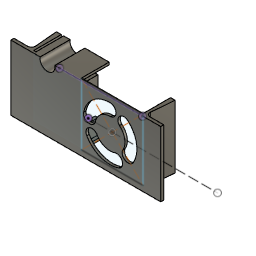
Tapa_fuente (Autodesk Fusion 360 design; units mm, degrees)
Autodesk Fusion 360 part; units mm, degrees
note: some values were not read from the file. Set by a fixed rule: which sketch regions a step uses.
sketch "Sketch1" plane through (0, 0, 0) normal (0, 1, 0) x (1, 0, 0)
  line L0 (38, -21) -> (-38, -21)
  line L1 (-38, -21) -> (-38, 21)
  line L2 (-38, 21) -> (38, 21)
  line L3 (38, 21) -> (38, -21)
  line L4 (38, -21) -> (-38, 21) construction
  line L5 (-38, -21) -> (38, 21) construction
  line L6 (-38, -21) -> (-50, -21)
  line L7 (-50, -21) -> (-50, 21)
  line L8 (-50, 21) -> (-38, 21)
  line L9 (-38, 21) -> (-38, -21)
  line L10 (38, -21) -> (50, -21)
  line L11 (50, -21) -> (50, 21)
  line L12 (50, 21) -> (38, 21)
  line L13 (38, 21) -> (38, -21)
  line L14 (-50, 21) -> (50, 21)
  line L15 (50, 21) -> (50, 22.5)
  line L16 (50, 22.5) -> (-50, 22.5)
  line L17 (-50, 22.5) -> (-50, 21)
  line L18 (36.5, -19.5) -> (-36.5, -19.5)
  line L19 (-36.5, -19.5) -> (-36.5, 19.5)
  line L20 (-36.5, 19.5) -> (36.5, 19.5)
  line L21 (36.5, 19.5) -> (36.5, -19.5)
  dimension "d1" = 42
  dimension "d2" = 76
  dimension "d3" = 12
  dimension "d4" = 12
  dimension "d5" = 1.5
  dimension "d10" = 1.5
  constraint horizontal L0
  constraint perpendicular L0 L1
  constraint parallel L0 L2
  constraint parallel L1 L3
  constraint coincident L4 origin
  constraint coincident L5 origin
  constraint horizontal L6
  constraint vertical L7
  constraint horizontal L8
  constraint vertical L9
  constraint horizontal L10
  constraint vertical L11
  constraint horizontal L12
  constraint vertical L13
  constraint horizontal L14
  constraint vertical L15
  constraint horizontal L16
  constraint vertical L17
  constraint collinear L11 L15
  measures "d1" distance of L0.end L1.end
  measures "d2" distance of L0.start L0.end
  measures "d3" distance of L0.end L6.end
  measures "d4" distance of L0.start L10.end
  measures "d5" distance of L7.end L16.end
extrude "Extrude1" add sketch "Sketch1" along normal blind 20 contours L0 L1 L2 L3 L9 L13 L14
extrude "Extrude2" add sketch "Sketch1" along normal blind 2 contours L3 L10 L11 L12 L13 L14 | L1 L6 L7 L8 L9 L14 | L2 L8 L12 L14 L15 L16 L17
extrude "Extrude3" add sketch "Sketch1" along normal blind 2 contours L18 L19 L20 L21
sketch "Sketch3" plane through (0, 2, 0) normal (0, 1, 0) x (-1, 0, 0)
  line L0 (-36.5, -19.5) -> (36.5, -19.5)
  line L1 (36.5, -19.5) -> (36.5, 19.5)
  line L2 (36.5, 19.5) -> (-36.5, 19.5)
  line L3 (-36.5, 19.5) -> (-36.5, -19.5)
extrude "Extrude4" add sketch "Sketch3" along normal up to surface (18 mm away)
sketch "Sketch4" plane through (0, 0, 0) normal (0, 1, 0) x (1, 0, 0)
  circle A0 centre (-25.5773, -20.0315) radius 5
  dimension "d15" = 10
  measures "d15" diameter of A0
extrude "Extrude5" cut sketch "Sketch4" along normal blind 25
draft "Draft1" angle -5 neutral plane through (0, 2, 0) pull (0, 1, 0) 1 faces at (38, 8, -7)
draft "Draft2" angle -5 neutral plane through (0, 2, 0) pull (0, 1, 0) 1 faces at (-38, 8, 7)
shell "Shell1" thickness 1.6 removed faces 1 at (-7.6005, 20, -8.7091)
sketch "Sketch6" plane through (0, 1.6, 0) normal (0, 1, 0) x (-1, 0, 0)
  line L0 (-36.3589, -19.4) -> (36.3589, -19.4)
  line L1 (36.3589, -19.4) -> (36.3589, 19.4)
  arc A0 (19.0076, 19.4) -> (32.147, 19.4) centre (25.5773, 20.0315) ccw
  line L2 (36.3589, 19.4) -> (32.147, 19.4)
  line L3 (-36.3589, 19.4) -> (-36.3589, -19.4)
  line L4 (0, 0) -> (-6.562, 0) construction
  line L5 (-6.562, 0) -> (-86.2837, 0) construction
  line L6 (4.4388, 20.5) -> (-36.5612, 20.5)
  line L7 (-36.5612, 20.5) -> (-36.5612, -20.5)
  line L8 (-36.5612, -20.5) -> (4.4388, -20.5)
  line L9 (4.4388, -20.5) -> (4.4388, 20.5)
  line L10 (4.4388, 20.5) -> (-36.5612, -20.5) construction
  line L11 (-36.5612, 20.5) -> (4.4388, -20.5) construction
  line L12 (19.0076, 19.4) -> (-36.3589, 19.4)
  point P0 (-16.0612, 0)
  dimension "d27" = 41
  dimension "d28" = 41
  constraint coincident L4.start origin
  constraint horizontal L4
  constraint parallel L4 L5
  constraint horizontal L6
  constraint perpendicular L6 L7
  constraint parallel L6 L8
  constraint parallel L7 L9
  constraint coincident L10 P0
  constraint coincident L11 P0
  constraint coincident L5 P0
  measures "d27" distance of L7.end L8.end
  measures "d28" distance of L6.end L7.end
extrude "Extrude6" cut sketch "Sketch6" along normal blind 130 contours L0 L3 L9 L12 | L0 L3 L6 L7 L8 L9 L12
sketch "Sketch7" plane through (0, 0, 0) normal (0, 0, 1) x (1, 0, 0)
sketch "Sketch8" plane through (0, 1.6, 0) normal (0, 1, 0) x (-1, 0, 0)
  line L0 (4.4388, 19.4) -> (4.4388, 20.5)
  line L1 (4.4388, 20.5) -> (-36.5612, 20.5)
  line L2 (-36.5612, 20.5) -> (-36.5612, -20.5)
  line L3 (-36.5612, -20.5) -> (4.4388, -20.5)
  line L4 (4.4388, -20.5) -> (4.4388, -19.4)
  line L5 (4.4388, -19.4) -> (36.3589, -19.4)
  line L6 (36.3589, -19.4) -> (36.3589, 19.4)
  arc A0 (19.0076, 19.4) -> (32.147, 19.4) centre (25.5773, 20.0315) ccw
  line L7 (36.3589, 19.4) -> (32.147, 19.4)
  line L8 (0, 0) -> (-84.2922, 0) construction
  circle A1 centre (-16.1448, 0) radius 10
  line L9 (-16.1448, 0) -> (-16.1448, 17.0215) construction
  arc A2 (1.4322, 3.6075) -> (-16.1448, 17.9434) centre (-16.1448, 0) ccw
  arc A3 (-6.3876, 2.0025) -> (1.4322, 3.6075) centre (-2.4777, 2.805) ccw
  arc A4 (-6.3876, 2.0025) -> (-16.1448, 9.9606) centre (-16.1448, 0) ccw
  arc A5 (-16.1448, 17.9434) -> (-16.1448, 9.9606) centre (-16.1448, 13.952) ccw
  arc A6 (-2.4777, 2.805) -> (-16.1448, 13.952) centre (-16.1448, 0) ccw construction
  arc A7 (-28.0575, 13.4184) -> (-31.6843, -8.9717) centre (-16.1448, 0) ccw
  arc A8 (-31.6843, -8.9717) -> (-24.7709, -4.9803) centre (-28.2276, -6.976) ccw
  arc A9 (-22.7576, 7.4487) -> (-24.7709, -4.9803) centre (-16.1448, 0) ccw
  arc A10 (-22.7576, 7.4487) -> (-28.0575, 13.4184) centre (-25.4076, 10.4336) ccw
  arc A11 (-21.8092, -17.0259) -> (-0.6054, -8.9717) centre (-16.1448, 0) ccw
  arc A12 (-0.6054, -8.9717) -> (-7.5187, -4.9803) centre (-4.062, -6.976) ccw
  arc A13 (-19.2892, -9.4512) -> (-7.5187, -4.9803) centre (-16.1448, 0) ccw
  arc A14 (-19.2892, -9.4512) -> (-21.8092, -17.0259) centre (-20.5492, -13.2386) ccw
  line L10 (19.0076, 19.4) -> (4.4388, 19.4)
  dimension "d31" = 20
  dimension "d33" = 360
  constraint coincident L8.start origin
  constraint horizontal L8
  constraint coincident L8 A1.centre
  constraint coincident A1.centre L9.start
  constraint perpendicular L8 L9
  constraint tangent A2 A3
  constraint tangent A3 A4
  constraint tangent A4 A5
  constraint tangent A2 A5
  constraint coincident L9 A5.centre
  measures "d31" diameter of A1
extrude "Extrude7" cut sketch "Sketch8" against normal blind 15 contours A1 A2 A3 A5 | A1 A11 A12 A14 | A1 A7 A8 A10
sketch "Sketch9" plane through (0, 1.6, 0) normal (0, 1, 0) x (-1, 0, 0)
  line L0 (4.4622, 17.4322) -> (6.4622, 17.4322)
  line L1 (6.4622, 17.4322) -> (6.4622, 7.4322)
  line L2 (6.4622, 7.4322) -> (4.4622, 7.4322)
  line L3 (4.4622, 7.4322) -> (4.4622, 17.4322)
  line L4 (-16.0432, 0.0175) -> (9.0898, 0.0175) construction
  line L5 (4.4622, -17.3972) -> (6.4622, -17.3972)
  line L6 (6.4622, -17.3972) -> (6.4622, -7.3972)
  line L7 (6.4622, -7.3972) -> (4.4622, -7.3972)
  line L8 (4.4622, -7.3972) -> (4.4622, -17.3972)
  dimension "d36" = 2
  dimension "d37" = 10
  constraint horizontal L0
  constraint vertical L1
  constraint horizontal L2
  constraint vertical L3
  constraint horizontal L4
  constraint symmetric L0.start L4 L5.start
  constraint symmetric L0.end L4 L5.end
  constraint symmetric L1.end L4 L6.end
  constraint symmetric L2.end L4 L7.end
  measures "d36" distance of L0.start L0.end
  measures "d37" distance of L0.start L2.end
extrude "Extrude8" add sketch "Sketch9" along normal blind 11
sketch "Sketch13" plane through (0, 20, 0) normal (0, 1, 0) x (-1, 0, 0)
  arc A0 (20.672, 21) -> (30.4826, 21) centre (25.5773, 20.0315) ccw
  line L0 (20.672, 21) -> (-39.5748, 21)
  line L1 (-39.5748, 21) -> (-39.5748, -21)
  line L2 (-39.5748, -21) -> (39.5748, -21)
  line L3 (39.5748, -21) -> (39.5748, 21)
  line L4 (39.5748, 21) -> (30.4826, 21)
  line L5 (-36.5612, 19.4) -> (-36.5612, 20.5)
  line L6 (-36.5612, 20.5) -> (4.4388, 20.5)
  line L7 (4.4388, 20.5) -> (4.4388, 19.4)
  line L8 (4.4388, 19.4) -> (19.0076, 19.4)
  arc A1 (19.0076, 19.4) -> (32.147, 19.4) centre (25.5773, 20.0315) ccw
  line L9 (32.147, 19.4) -> (37.9687, 19.4)
  line L10 (37.9687, 19.4) -> (37.9687, -19.4)
  line L11 (37.9687, -19.4) -> (4.4388, -19.4)
  line L12 (4.4388, -19.4) -> (4.4388, -20.5)
  line L13 (4.4388, -20.5) -> (-36.5612, -20.5)
  line L14 (-36.5612, -20.5) -> (-36.5612, -19.4)
  line L15 (-36.5612, -19.4) -> (-37.9687, -19.4)
  line L16 (-37.9687, -19.4) -> (-37.9687, 19.4)
  line L17 (-37.9687, 19.4) -> (-36.5612, 19.4)
  line L18 (-36.5612, 23.0341) -> (4.4712, 23.0341)
  line L19 (4.4712, 23.0341) -> (4.4712, -29.06)
  line L20 (4.4712, -29.06) -> (-36.5612, -29.06)
  line L21 (-36.5612, -29.06) -> (-36.5612, 23.0341)
  line L22 (36.3303, 21.4138) -> (34.8169, 21.4138)
  line L23 (34.8169, 21.4138) -> (34.8169, -30.2947)
  line L24 (34.8169, -30.2947) -> (36.3303, -30.2947)
  line L25 (36.3303, -30.2947) -> (36.3303, 21.4138)
  constraint horizontal L18
  constraint vertical L19
  constraint horizontal L20
  constraint vertical L21
  constraint horizontal L22
  constraint vertical L23
  constraint horizontal L24
  constraint vertical L25
extrude "Extrude12" cut sketch "Sketch13" against normal up to surface (18.4 mm away) contours L0 L6 L7 L8 L19 L21 | L4 L9 L23 L25 | L2 L11 L12 L13 L19 L21 | L2 L11 L23 L25
fillet "Fillet1" radius 2.5 2 edges at (-6.4622, 1.6, 12.4322) (-6.4622, 1.6, -12.3972)
fillet "Fillet2" radius 2.5 2 edges at (-38, 2, 0) (38, 2, 0)
fillet "Fillet3" radius 2 3 edges at (-11.7394, 1.6, 19.4) (-25.5773, 1.6, 13.4315) (-19.6441, 1.6, -19.4)
